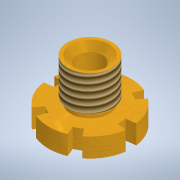
# Autodesk Inventor part: Part31
Saved by Autodesk Inventor 2020 (Build 240168000, 168)
## iProperties
Created: 2021-10-26
Part Number: Part31
Material: Brass, Soft Yellow, Welded
Document SubType Name: Modeling
Designer: simon.erikssonwestl
Density: 8.5 g/cm^3
Appearance: Weld - Brass
Author: simon.erikssonwestl
Autodesk Inventor part; units mm, degrees
ref_plane "YZ Plane" through (0, 0, 0) normal (1, 0, 0) x (0, 1, 0)
ref_plane "XZ Plane" through (0, 0, 0) normal (0, 1, 0) x (-1, 0, 0)
ref_plane "XY Plane" through (0, 0, 0) normal (0, 0, 1) x (1, 0, 0)
sketch "Sketch1" plane through (0, 0, 0) normal (0, 1, 0) x (-1, 0, 0)
  circle A0 centre (0, 0) radius 6.5
  arc A1 (4.9572, -0.6526) -> (4.9572, 0.6526) centre (0, 0) ccw
  line L0 (6.5, 0) -> (0, 0)
  line L1 (4.9572, -0.6526) -> (6.4979, -0.8555)
  line L2 (4.9572, 0.6526) -> (6.9401, 0.9137)
  line L3 (0, 0) -> (7, 0) construction
  line L4 (3.0438, 3.9668) -> (3.9898, 5.1996)
  arc A2 (3.0438, 3.9668) -> (1.9134, 4.6194) centre (0, 0) ccw
  line L5 (1.9134, 4.6194) -> (2.6788, 6.4672)
  line L6 (-1.9134, 4.6194) -> (-2.5081, 6.0551)
  arc A3 (-1.9134, 4.6194) -> (-3.0438, 3.9668) centre (0, 0) ccw
  line L7 (-3.0438, 3.9668) -> (-4.2613, 5.5535)
  line L8 (-4.9572, 0.6526) -> (-6.4979, 0.8555)
  arc A4 (-4.9572, 0.6526) -> (-4.9572, -0.6526) centre (0, 0) ccw
  line L9 (-4.9572, -0.6526) -> (-6.9401, -0.9137)
  line L10 (-3.0438, -3.9668) -> (-3.9898, -5.1996)
  arc A5 (-3.0438, -3.9668) -> (-1.9134, -4.6194) centre (0, 0) ccw
  line L11 (-1.9134, -4.6194) -> (-2.6788, -6.4672)
  line L12 (1.9134, -4.6194) -> (2.5081, -6.0551)
  arc A6 (1.9134, -4.6194) -> (3.0438, -3.9668) centre (0, 0) ccw
  line L13 (3.0438, -3.9668) -> (4.2613, -5.5535)
  point P0 (-6.4444, -0.8484)
  point P1 (-3.9569, -5.1568)
  point P2 (-2.4874, -6.0052)
  point P3 (2.4874, -6.0052)
  point P4 (3.9569, -5.1568)
  point P5 (6.4444, -0.8484)
  point P6 (6.4444, 0.8484)
  point P7 (3.9569, 5.1568)
  point P8 (2.4874, 6.0052)
  point P9 (-2.4874, 6.0052)
  point P10 (-3.9569, 5.1568)
  point P11 (-6.4444, 0.8484)
  dimension "d0" = 13
  dimension "d1" = 10
  dimension "d2" = 6.554
  dimension "d3" = 7.5
  dimension "d4" = 7
  dimension "d5" = 7.5
  dimension "d8" = 360
  constraints: 28 end point, 12 point on circle, 6 centre point, 2 coincident, 2 horizontal, 52 other
  measures "d1" diameter of A1
  measures "d2" distance of L0.end L1.end
  measures "d3" angle of L1 L0
  measures "d4" distance of L0.end L2.end
  measures "d5" angle of L3 L2
extrude "Extrusion1" add sketch "Sketch1" along normal blind 3 contours L2 A1 L1 A0 L13 A6 L12 L11 A5 L10 L9 A4 L8 L7 A3 L6 L5 A2 L4
sketch "Sketch2" plane through (0, 3, 0) normal (0, 1, 0) x (1, 0, 0)
  arc A0 (-2.4874, -6.0052) -> (2.4874, -6.0052) centre (0, 0) ccw projected
  line L0 (2.4874, -6.0052) -> (1.9134, -4.6194) projected
  arc A1 (1.9134, -4.6194) -> (3.0438, -3.9668) centre (0, 0) ccw projected
  line L1 (3.0438, -3.9668) -> (3.9569, -5.1568) projected
  arc A2 (3.9569, -5.1568) -> (6.4444, -0.8484) centre (0, 0) ccw projected
  line L2 (6.4444, -0.8484) -> (4.9572, -0.6526) projected
  arc A3 (4.9572, -0.6526) -> (4.9572, 0.6526) centre (0, 0) ccw projected
  line L3 (4.9572, 0.6526) -> (6.4444, 0.8484) projected
  arc A4 (6.4444, 0.8484) -> (3.9569, 5.1568) centre (0, 0) ccw projected
  line L4 (3.9569, 5.1568) -> (3.0438, 3.9668) projected
  arc A5 (3.0438, 3.9668) -> (1.9134, 4.6194) centre (0, 0) ccw projected
  line L5 (1.9134, 4.6194) -> (2.4874, 6.0052) projected
  arc A6 (2.4874, 6.0052) -> (-2.4874, 6.0052) centre (0, 0) ccw projected
  line L6 (-2.4874, 6.0052) -> (-1.9134, 4.6194) projected
  arc A7 (-1.9134, 4.6194) -> (-3.0438, 3.9668) centre (0, 0) ccw projected
  line L7 (-3.0438, 3.9668) -> (-3.9569, 5.1568) projected
  arc A8 (-3.9569, 5.1568) -> (-6.4444, 0.8484) centre (0, 0) ccw projected
  line L8 (-6.4444, 0.8484) -> (-4.9572, 0.6526) projected
  arc A9 (-4.9572, 0.6526) -> (-4.9572, -0.6526) centre (0, 0) ccw projected
  line L9 (-4.9572, -0.6526) -> (-6.4444, -0.8484) projected
  arc A10 (-6.4444, -0.8484) -> (-3.9569, -5.1568) centre (0, 0) ccw projected
  line L10 (-3.9569, -5.1568) -> (-3.0438, -3.9668) projected
  arc A11 (-3.0438, -3.9668) -> (-1.9134, -4.6194) centre (0, 0) ccw projected
  line L11 (-1.9134, -4.6194) -> (-2.4874, -6.0052) projected
  circle A12 centre (0, 0) radius 3
  dimension "d12" = 6
  constraints: 1 centre point, 1 coincident
  measures "d12" diameter of A12
extrude "Extrusion2" add sketch "Sketch2" along normal blind 1 contours A12
sketch "Sketch3" plane through (0, 4, 0) normal (0, 1, 0) x (1, 0, 0)
  circle A0 centre (0, 0) radius 3.5
  dimension "d15" = 7
  constraints: 1 centre point, 1 coincident
  measures "d15" diameter of A0
extrude "Extrusion3" add sketch "Sketch3" along normal blind 5.5
sketch "Sketch4" plane through (0, 9.5, 0) normal (0, 1, 0) x (1, 0, 0)
  point P0 (0, 0)
  point P1 (0, 0)
  constraints: 1 coincident
hole "Hole1" at (0, 9.5, 0) direction (0, -1, 0) diameter 4 end through all countersink diameter 6 countersink angle 90
thread "Thread1" size "M7x1" class "6g" standard "ANSI Metric M Profile" length 10
body "Solid1"
